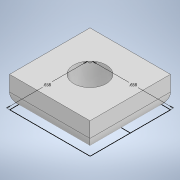
# Autodesk Inventor part: SquareRetainingClip
Saved by Autodesk Inventor 2020 (Build 240168000, 168)
## iProperties
Created: 2023-02-18
Part Number: SquareRetainingClip
Material: Generic
Document SubType Name: Modeling
Designer: Beaucage
Density: 1 g/cm^3
Appearance: Default
Author: Beaucage
Autodesk Inventor part; units mm, degrees
ref_plane "YZ Plane" through (0, 0, 0) normal (1, 0, 0) x (0, 1, 0)
ref_plane "XZ Plane" through (0, 0, 0) normal (0, 1, 0) x (-1, 0, 0)
ref_plane "XY Plane" through (0, 0, 0) normal (0, 0, 1) x (1, 0, 0)
sketch "Sketch1" plane through (0, 0, 0) normal (0, 1, 0) x (-1, 0, 0)
  line L0 (0, 0) -> (16.7132, 0)
  line L1 (16.7132, 0) -> (16.7132, -16.7132)
  line L2 (16.7132, -16.7132) -> (0, -16.7132)
  line L3 (0, -16.7132) -> (0, 0)
  line L4 (16.7132, 0) -> (16.7132, -8.3566)
  line L5 (16.7132, -16.7132) -> (8.2065, -16.7132)
  line L6 (0, 0) -> (0, -8.3566)
  line L7 (0, -8.3566) -> (16.7132, -8.3566)
  line L8 (16.7132, -8.3566) -> (8.3566, -8.3566)
  dimension "d0" = 16.7132
  dimension "d1" = 16.7132
  constraints: 18 end point, 3 midpoint, 2 parallel, 2 perpendicular, 1 horizontal, 1 point on line
  measures "d0" distance of L1.end L2.end
  measures "d1" distance of L0.end L1.end
extrude "Extrusion1" add sketch "Sketch1" along normal blind 6.35
hole "Hole1" at (-8.3566, 0, -8.3566) direction (0, 1, 0) diameter 6.7564 end through all counterbore diameter 11.1252 counterbore depth 1.5875 clearance for "Socket Head Cap Screw" size "1/4" standard "Ansi Unified Screw Threads"
fillet "Fillet1" radius 3.175 4 edges at (-8.3566, 0, 0) (-16.7132, 0, -8.3566) (0, 0, -8.3566) (-8.3566, 0, -16.7132)
body "Solid1"
